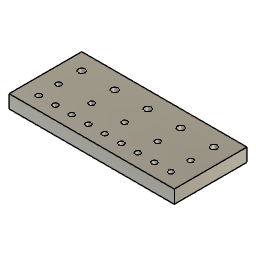
jig v1 (Autodesk Fusion 360 design; units mm, degrees)
Autodesk Fusion 360 part; units mm, degrees
sketch "スケッチ1" plane through (0, 0, 0) normal (0, 0, 1) x (1, 0, 0)
  line L0 (0, 0) -> (250, 0)
  line L1 (250, 0) -> (250, 110)
  line L2 (250, 110) -> (0, 110)
  line L3 (0, 110) -> (0, 0)
  circle A0 centre (25, 20) radius 4
  circle A1 centre (25, 85) radius 5
  circle A2 centre (75, 85) radius 5
  circle A3 centre (125, 85) radius 5
  circle A4 centre (175, 85) radius 5
  circle A5 centre (225, 85) radius 5
  circle A6 centre (50, 20) radius 4
  circle A7 centre (75, 20) radius 4
  circle A8 centre (100, 20) radius 4
  circle A9 centre (125, 20) radius 4
  circle A10 centre (150, 20) radius 4
  circle A11 centre (175, 20) radius 4
  circle A12 centre (200, 20) radius 4
  circle A13 centre (225, 20) radius 4
  circle A14 centre (75, 50) radius 4
  circle A15 centre (25, 50) radius 4
  circle A16 centre (125, 50) radius 4
  circle A17 centre (175, 50) radius 4
  circle A18 centre (225, 50) radius 4
  dimension "d1" = 110
  dimension "d2" = 250
  dimension "d3" = 8
  dimension "d4" = 10
  dimension "d7" = 50
  dimension "d8" = 0
  dimension "d11" = 25
  dimension "d12" = 0
  dimension "d15" = -30
  dimension "d16" = 30
  dimension "d17" = 25
  dimension "d18" = 25
  dimension "d19" = 20
  dimension "d20" = 25
  constraint horizontal L0
  constraint vertical L1
  constraint horizontal L2
  constraint vertical L3
  constraint coincident L0.start L3.end
  measures "d1" distance of L0.start L2.end
  measures "d2" distance of L0.start L0.end
  measures "d3" diameter of A0
  measures "d4" diameter of A1
  measures "d17" distance of L3 A1.centre
  measures "d18" distance of L3 A0.centre
  measures "d19" distance of L0 A0.centre
  measures "d20" distance of L2 A1.centre
extrude "押し出し1" add sketch "スケッチ1" along normal blind 20
